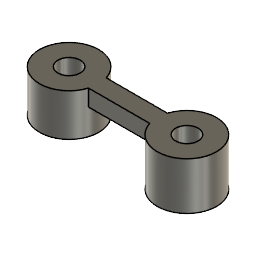
Linkers (Autodesk Fusion 360 design; units mm, degrees)
Autodesk Fusion 360 part; units mm, degrees
sketch "Sketch1" plane through (0, 0, 0) normal (0, 0, 1) x (1, 0, 0)
  circle A0 centre (0, 0) radius 4.5
  line L0 (0, 0) -> (17.87, 0) construction
  circle A1 centre (17.87, 0) radius 4.5
  line L1 (13.5773, 1.35) -> (4.2927, 1.35)
  line L2 (13.5773, -1.35) -> (4.2927, -1.35)
  dimension "d1" = 9
  dimension "d2" = 17.87
  dimension "d3" = 9
  dimension "d4" = 2.7
  dimension "d5" = 1.35
  constraint coincident A0.centre L0.start
  constraint horizontal L0
  constraint coincident L0.end A1.centre
  constraint coincident A1 L1.start
  constraint coincident A0 L1.end
  constraint horizontal L1
  constraint coincident A1 L2.start
  constraint coincident A0 L2.end
  constraint parallel L0 L2
  measures "d1" diameter of A0
  measures "d2" distance of A0.centre L0.end
  measures "d3" diameter of A1
  measures "d4" distance of L1 L2
  measures "d5" distance of L0 L1
extrude "Extrude1" add sketch "Sketch1" along normal blind 6.4 contours A0 makes body 1
sketch "Sketch2" plane through (0, 0, 6.4) normal (0, 0, 1) x (-1, 0, 0)
  circle A0 centre (0, 0) radius 4.5
  line L0 (0, 0) -> (-17.87, 0) construction
  circle A1 centre (-17.87, 0) radius 4.5
  dimension "d8" = 17.87
  dimension "d9" = 9
  constraint coincident A0.centre L0.start
  constraint horizontal L0
  constraint coincident L0.end A1.centre
  measures "d8" distance of A0.centre L0.end
  measures "d9" diameter of A1
extrude "Extrude2" add sketch "Sketch2" against normal blind 7.2 separate body contours A1 makes body 2
sketch "Sketch3" plane through (0, 0, 6.4) normal (0, 0, 1) x (-1, 0, 0)
  circle A0 centre (0, 0) radius 4.5
  circle A1 centre (0, 0) radius 4.5
  line L0 (0, 0) -> (-17.87, 0) construction
  circle A2 centre (-17.87, 0) radius 4.5
  line L1 (-4.2925, -1.3507) -> (-13.5775, -1.3507)
  line L2 (-13.5775, 1.3507) -> (-4.2925, 1.3507)
  dimension "d12" = 17.87
  dimension "d13" = 9
  dimension "d14" = 9.285
  dimension "d15" = 9.285
  constraint coincident A0.centre A1.centre
  constraint horizontal L0
  constraint coincident L0.end A2.centre
  constraint coincident A1 L1.start
  constraint coincident A2 L1.end
  constraint parallel L0 L1
  constraint coincident A2 L2.start
  constraint coincident A1 L2.end
  constraint horizontal L2
  measures "d12" distance of A0.centre L0.end
  measures "d13" diameter of A2
  measures "d14" distance of L1.start L1.end
  measures "d15" distance of L2.start L2.end
extrude "Extrude3" add sketch "Sketch3" against normal blind 2.49 contours A0 A1 A2 L1 L2 bodies 1 2
sketch "Sketch4" plane through (0, 0, 0) normal (0, 1, 0) x (1, 0, 0)
hole "Hole1" at (0, 0, 6.4) direction (0, 0, -1) diameter 3.4 depth 7 tip angle 118 bodies 1
hole "Hole2" at (17.87, 0, 6.4) direction (0, 0, -1) diameter 3.4 depth 7 tip angle 118 bodies 1
